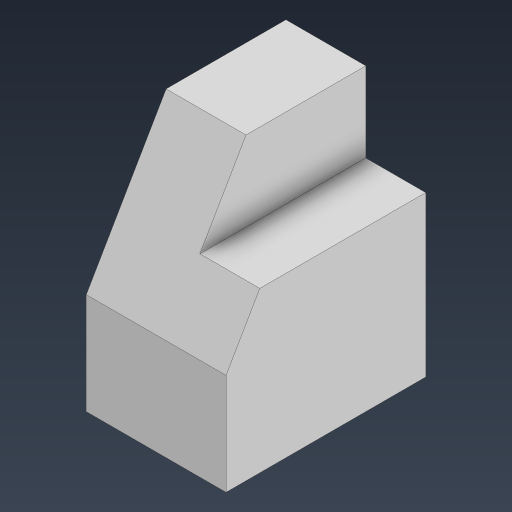
# Autodesk Inventor part: 3D Model
Saved by Autodesk Inventor 2024 (Build 280153000, 153)
## iProperties
Created: 2024-03-05
Part Number: 3D Model
Material: Genérico
Document SubType Name: Modeling
Designer: Administrator
Density: 1 g/cm^3
Appearance: Padrão
Author: Administrator
Autodesk Inventor part; units mm, degrees
ref_plane "YZ Plane" through (0, 0, 0) normal (1, 0, 0) x (0, 1, 0)
ref_plane "XZ Plane" through (0, 0, 0) normal (0, 1, 0) x (-1, 0, 0)
ref_plane "XY Plane" through (0, 0, 0) normal (0, 0, 1) x (1, 0, 0)
sketch "Esboço1" plane through (0, 0, 0) normal (0, 1, 0) x (-1, 0, 0)
  line L0 (17.5, -25) -> (-17.5, -25)
  line L1 (-17.5, -25) -> (-17.5, 25)
  line L2 (-17.5, 25) -> (17.5, 25)
  line L3 (17.5, 25) -> (17.5, -25)
  line L4 (17.5, -25) -> (-17.5, 25) construction
  line L5 (-17.5, -25) -> (17.5, 25) construction
  point P0 (0, 0)
  dimension "d0" = 35
  dimension "d1" = 50
  constraints: 12 end point, 2 midpoint, 2 parallel, 1 horizontal, 1 perpendicular
  measures "d0" distance of L1.end L2.end
  measures "d1" distance of L0.end L1.end
extrude "Extrusão1" add sketch "Esboço1" along normal blind 60
chamfer "Chanfro1" distance 20 angle 60 1 edges at (0, 60, 25) measured on face at (5.8333, 60, 8.3333)
sketch "Esboço2" plane through (17.5, 0, -25) normal (0, 0, -1) x (-1, 0, 0)
  line L0 (0, 60) -> (15, 60)
  line L1 (15, 60) -> (15, 40)
  line L2 (15, 40) -> (0, 40)
  line L3 (0, 40) -> (0, 60)
  line L4 (35, 0) -> (35, 60) projected
  line L5 (0, 0) -> (35, 0) projected
  point P0 (17.5, 0)
  dimension "d7" = 20
  dimension "d8" = 40
  constraints: 8 end point, 2 parallel, 1 coincident, 1 horizontal, 1 perpendicular
  measures "d7" distance between parallel lines of L4 L1
  measures "d8" distance between parallel lines of L5 L2
extrude "Extrusão2" cut sketch "Esboço2" against normal through all
